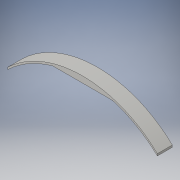
# Autodesk Inventor part: ClipBottom
Saved by Autodesk Inventor 2016 (Build 200138000, 138)
## iProperties
Created: 2016-08-20
Part Number: ClipBottom
Material: Generic
Document SubType Name: Modeling
Designer: yash
Density: 1 g/cm^3
Appearance: Default
Author: yash
Autodesk Inventor part; units mm, degrees
ref_plane "YZ Plane" through (0, 0, 0) normal (1, 0, 0) x (0, 1, 0)
ref_plane "XZ Plane" through (0, 0, 0) normal (0, 1, 0) x (-1, 0, 0)
ref_plane "XY Plane" through (0, 0, 0) normal (0, 0, 1) x (1, 0, 0)
sketch "Sketch1" plane through (0, 0, 0) normal (0, 0, 1) x (1, 0, 0)
  line L0 (0, 0) -> (127, 0) construction
  line L1 (0, 0) -> (63.5, 0) construction
  line L2 (63.5, 0) -> (63.5, 25.4) construction
  line L3 (0, 0) -> (0, 1.7272)
  line L4 (127, 0) -> (127, 1.7272)
  line L5 (63.5, 25.4) -> (63.5, 27.1272)
  line L6 (63.5, 25.4) -> (65.2272, 25.4) construction
  arc A0 (127, 1.7272) -> (0, 1.7272) centre (63.5, -64.9478) ccw
  line L7 (38.1, 21.8272) -> (88.9, 21.8272)
  arc A1 (127, 0) -> (88.9, 21.8272) centre (63.5, -66.675) ccw
  arc A2 (38.1, 21.8272) -> (0, 0) centre (63.5, -66.675) ccw
  dimension "d0" = 127
  dimension "d1" = 63.5
  dimension "d2" = 25.4
  dimension "d3" = 1.7272
  dimension "d4" = 1.7272
  dimension "d5" = 1.7272
  dimension "d6" = 90
  dimension "d8" = 50.8
  constraints: 16 end point, 7 point on circle, 3 centre point, 3 horizontal, 3 vertical, 2 perpendicular, 1 equal radius, 1 midpoint, 1 tangent
  measures "d0" distance of L0.start L0.end
  measures "d1" distance of L0.start L1.end
  measures "d2" distance of L1.end L2.end
  measures "d3" distance of L0.start L3.end
  measures "d4" distance of L0.end L4.end
  measures "d5" distance of L2.end L5.end
  measures "d6" angle of L6 L5
  measures "d8" distance of L7.end L7.start
extrude "Extrusion1" add sketch "Sketch1" along normal blind 12.7
body "Solid1"
